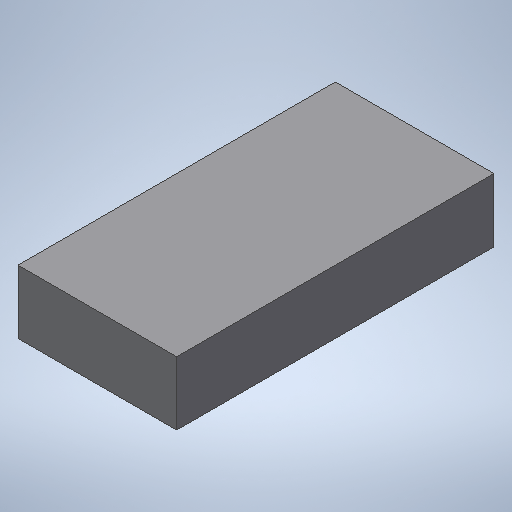
# Autodesk Inventor part: Part1-01
Saved by Autodesk Inventor 2027 (Build 310192060, 192F)
## iProperties
Created: 2026-06-21
Part Number: Part1-01
Material: Generisch
Document SubType Name: Modeling
Designer: tobia
Density: 1 g/cm^3
Appearance: Vorgabe
Author: tobia
Autodesk Inventor part; units mm, degrees
ref_plane "YZ Plane" through (0, 0, 0) normal (1, 0, 0) x (0, 1, 0)
ref_plane "XZ Plane" through (0, 0, 0) normal (0, 1, 0) x (-1, 0, 0)
ref_plane "XY Plane" through (0, 0, 0) normal (0, 0, 1) x (1, 0, 0)
sketch "Sketch1" plane through (0, 0, 0) normal (0, 1, 0) x (-1, 0, 0)
  line L0 (-12.5, -25) -> (12.5, -25)
  line L1 (12.5, -25) -> (12.5, 25)
  line L2 (12.5, 25) -> (-12.5, 25)
  line L3 (-12.5, 25) -> (-12.5, -25)
  line L4 (-12.5, -25) -> (12.5, 25) construction
  line L5 (12.5, -25) -> (-12.5, 25) construction
  point P0 (0, 0)
  dimension "Width" = 25
  dimension "Length" = 50
  constraints: 12 end point, 2 midpoint, 2 parallel, 1 horizontal, 1 perpendicular
  measures "Width" distance of L2.end L1.end
  measures "Length" distance of L0.end L1.end
extrude "Extrusion1" add sketch "Sketch1" along normal blind 10
body "Solid1"
